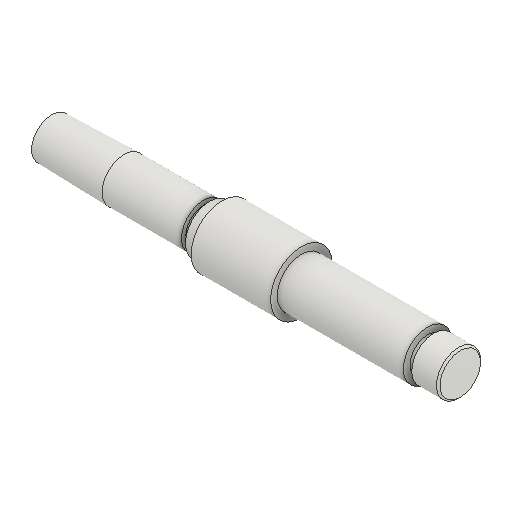
# Autodesk Inventor part: Вал
Saved by Autodesk Inventor 2021 (Build 250183000, 183)
## iProperties
CustomPartVersion: 1
Created: 2021-09-09
Part Number: Вал
Material: Steel
Document SubType Name: Modeling
Designer: Dison
Density: 1 g/cm^3
Appearance: Steel
Length: 463,000 мм
Author: Dison
Autodesk Inventor part; units mm, degrees
ref_plane "Начальная плоскость" through (0, 0, 0) normal (1, 0, 0) x (0, 1, 0)
ref_plane "XZ Plane" through (0, 0, 0) normal (0, 1, 0) x (-1, 0, 0)
ref_plane "XY Plane" through (0, 0, 0) normal (0, 0, 1) x (1, 0, 0)
sketch "Основной эскиз" plane through (0, 0, 0) normal (0, 0, 1) x (1, 0, 0)
  line L0 (0, 0) -> (463, 0)
  line L1 (0, 0) -> (0, 22.95)
  line L2 (0, 22.95) -> (82, 25)
  line L3 (172, 25) -> (172, 20)
  line L4 (82, 25) -> (172, 25)
  line L5 (172, 20) -> (179, 20)
  line L6 (179, 20) -> (179, 27.5)
  line L7 (179, 27.5) -> (193, 27.5)
  line L8 (193, 27.5) -> (193, 35)
  line L9 (283, 35) -> (283, 27.5)
  line L10 (193, 35) -> (283, 35)
  line L11 (426, 27.5) -> (426, 20)
  line L12 (283, 27.5) -> (426, 27.5)
  line L13 (426, 20) -> (433, 20)
  line L14 (433, 20) -> (433, 25)
  line L15 (463, 25) -> (463, 0)
  line L16 (433, 25) -> (463, 25)
  dimension "d3" = 50
  dimension "d4" = 40
  dimension "d5" = 55
  dimension "d6" = 70
  dimension "d7" = 55
  dimension "d8" = 40
  dimension "d9" = 50
  constraints: 34 end point, 8 vertical, 1 horizontal
  measures "d3" diameter of L4 L0
  measures "d4" diameter of L5 L0
  measures "d5" diameter of L7 L0
  measures "d6" diameter of L10 L0
  measures "d7" diameter of L12 L0
  measures "d8" diameter of L13 L0
  measures "d9" diameter of L16 L0
revolve "Вращение1" add sketch "Основной эскиз" angle 360 about axis through (0, 0, 0) along (1, 0, 0)
chamfer "Фаска1" distance 2 angle 45 1 edges at (463, -25, 0) measured on face at (462.5, -25, 0)
equation "\"Length\" = 463"
